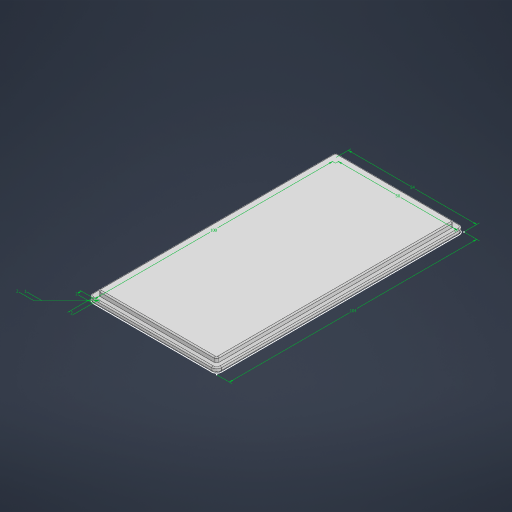
# Autodesk Inventor part: connection box lid
Saved by Autodesk Inventor 2024.2 (Build 282272000, 272)
## iProperties
Created: 2025-07-03
Part Number: connection box lid
Material: Generic
Document SubType Name: Modeling
Designer: Moe
Density: 1 g/cm^3
Appearance: Default
Author: Moe
Autodesk Inventor part; units mm, degrees
ref_plane "YZ Plane" through (0, 0, 0) normal (1, 0, 0) x (0, 1, 0)
ref_plane "XZ Plane" through (0, 0, 0) normal (0, 1, 0) x (-1, 0, 0)
ref_plane "XY Plane" through (0, 0, 0) normal (0, 0, 1) x (1, 0, 0)
sketch "Sketch1" plane through (0, 0, 0) normal (0, 1, 0) x (-1, 0, 0)
  line L0 (1, 0) -> (49, 0)
  line L1 (50, -1) -> (50, -99)
  line L2 (49, -100) -> (1, -100)
  line L3 (0, -99) -> (0, -1)
  line L4 (50, 2) -> (0, 2)
  line L5 (-2, 0) -> (-2, -100)
  line L6 (0, -102) -> (50, -102)
  line L7 (52, -100) -> (52, 0)
  arc A0 (52, 0) -> (50, 2) centre (50, 0) ccw
  arc A1 (0, 2) -> (-2, 0) centre (0, 0) ccw
  arc A2 (-2, -100) -> (0, -102) centre (0, -100) ccw
  arc A3 (50, -102) -> (52, -100) centre (50, -100) ccw
  arc A4 (50, -1) -> (49, 0) centre (49, -1) ccw
  arc A5 (1, 0) -> (0, -1) centre (1, -1) ccw
  arc A6 (0, -99) -> (1, -100) centre (1, -99) ccw
  arc A7 (49, -100) -> (50, -99) centre (49, -99) ccw
  point P0 (0, 0)
  point P1 (50, -100)
  point P2 (50, 0)
  point P3 (0, -100)
  point P4 (-2, -102)
  point P5 (-2, 2)
  point P6 (52, -102)
  dimension "d0" = 50
  dimension "d1" = 100
  dimension "d2" = 54
  dimension "d3" = 104
  dimension "d4" = 2
  dimension "d5" = 2
  dimension "d6" = 2
  dimension "d7" = 1
  constraints: 16 end point, 16 point on circle, 16 tangent, 14 point on line, 8 centre point, 6 equal radius, 4 parallel, 2 horizontal, 2 perpendicular
  measures "d0" distance of point (50, -100) point (0, -100)
  measures "d1" distance of point (50, 0) point (50, -100)
  measures "d2" distance of point (52, -102) point (-2, -102)
  measures "d3" distance of point (-2, -102) point (-2, 2)
  measures "d4" distance between parallel lines of L7 L1
  measures "d5" distance between parallel lines of L4 L0
  measures "d6" radius of A0
  measures "d7" radius of A4
extrude "Extrusion1" add sketch "Sketch1" along normal blind 4 contours L0 A4 L1 A7 L2 A6 L3 A5
extrude "Extrusion2" add sketch "Sketch1" along normal blind 2
fillet "Fillet1" radius 0.5 24 edges at (-0.2929, 4, -0.2929) (0, 4, -50) (-0.2929, 4, -99.7071) (-25, 4, -100) (-49.7071, 4, -99.7071) (-50, 4, -50) (-49.7071, 4, -0.2929) (-25, 4, 0) (1.4142, 2, 1.4142) (2, 2, -50) (1.4142, 2, -101.4142) (-25, 2, -102) (-51.4142, 2, -101.4142) (-52, 2, -50) (-51.4142, 2, 1.4142) (-25, 2, 2) (1.4142, 0, 1.4142) (2, 0, -50) (1.4142, 0, -101.4142) (-25, 0, -102) (-51.4142, 0, -101.4142) (-52, 0, -50) (-51.4142, 0, 1.4142) (-25, 0, 2)
body "Solid1"
